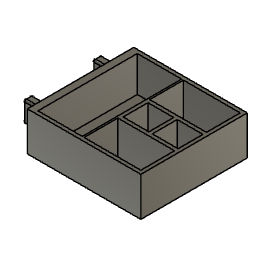
NP FW50 Charge Storagetray upright v4 (Autodesk Fusion 360 design; units mm, degrees)
Autodesk Fusion 360 part; units mm, degrees
note: some values were not read from the file. Chosen so that the rebuilt part matches the saved one: which face or edge a step refers to.
sketch "Skizze1" plane through (0, 0, 0) normal (0, 0, 1) x (1, 0, 0)
  line L0 (0, 0) -> (62, 0)
  line L1 (62, 0) -> (62, 60)
  line L2 (62, 60) -> (0, 60)
  line L3 (0, 60) -> (0, 0)
  line L4 (60, 2) -> (60, 58)
  line L5 (60, 58) -> (2, 58)
  line L6 (2, 58) -> (2, 2)
  line L7 (2, 2) -> (60, 2)
  line L8 (2, 58) -> (27, 58)
  line L9 (27, 58) -> (27, 2)
  line L10 (27, 2) -> (2, 2)
  line L11 (2, 2) -> (2, 58)
  line L12 (60, 58) -> (28, 58)
  line L13 (28, 58) -> (28, 39)
  line L14 (28, 39) -> (60, 39)
  line L15 (60, 39) -> (60, 58)
  line L16 (60, 2) -> (28, 2)
  line L17 (28, 2) -> (28, 21)
  line L18 (28, 21) -> (60, 21)
  line L19 (60, 21) -> (60, 2)
  line L20 (0, 60) -> (-2, 60)
  line L21 (-2, 60) -> (-2, 0)
  line L22 (-2, 0) -> (0, 0)
  line L23 (0, 0) -> (0, 60)
  dimension "d1" = 62
  dimension "d2" = 60
  dimension "d3" = -2
  dimension "d4" = 25
  dimension "d5" = 56
  dimension "d6" = 32
  dimension "d7" = 19
  dimension "d8" = 32
  dimension "d9" = 19
  dimension "d14" = 2
  dimension "d15" = 60
  constraint horizontal L0
  constraint vertical L1
  constraint horizontal L2
  constraint vertical L3
  constraint coincident L0.start L3.end
  constraint horizontal L8
  constraint vertical L9
  constraint horizontal L10
  constraint vertical L11
  constraint horizontal L12
  constraint vertical L13
  constraint horizontal L14
  constraint vertical L15
  constraint horizontal L16
  constraint vertical L17
  constraint horizontal L18
  constraint vertical L19
  constraint horizontal L20
  constraint vertical L21
  constraint horizontal L22
  constraint vertical L23
  measures "d1" distance of L0.start L0.end
  measures "d2" distance of L0.start L2.end
  measures "d4" distance of L5.end L8.end
  measures "d5" distance of L5.end L6.end
  measures "d6" distance of L4.end L12.end
  measures "d7" distance of L4.end L14.end
  measures "d8" distance of L4.start L16.end
  measures "d9" distance of L4.start L18.end
  measures "d14" distance of L2.end L20.end
  measures "d15" distance of L2.end L0.start
extrude "Extrusion1" add sketch "Skizze1" along normal blind 20 contours L0 L1 L2 L3 L23 | L3 L20 L21 L22 L23 | L4 L5 L7 L9 L13 L14 L17 L18
extrude "Extrusion2" add sketch "Skizze1" against normal blind 2 contours L0 L1 L2 L3 L23 | L3 L20 L21 L22 L23 | L4 L7 L16 L17 L18 L19 | L4 L5 L7 L9 L13 L14 L17 L18 | L4 L5 L12 L13 L14 L15 | L5 L6 L7 L8 L9 L10 L11
sketch "Skizze2" plane through (0, 0, 20) normal (0, 0, 1) x (-1, 0, 0)
  line L0 (-60, -58) -> (-60, -39)
  line L1 (-60, -39) -> (-28, -39)
  line L2 (-28, -39) -> (-28, -58)
  line L3 (-28, -58) -> (-60, -58)
  line L4 (-28, -21) -> (-60, -21)
  line L5 (-60, -21) -> (-60, -2)
  line L6 (-60, -2) -> (-28, -2)
  line L7 (-28, -2) -> (-28, -21)
  line L8 (-27, -2) -> (-2, -2)
  line L9 (-2, -2) -> (-2, -58)
  line L10 (-2, -58) -> (-27, -58)
  line L11 (-27, -58) -> (-27, -2)
  line L12 (2, 0) -> (-62, 0)
  line L13 (-62, 0) -> (-62, -60)
  line L14 (-62, -60) -> (2, -60)
  line L15 (2, -60) -> (2, 0)
  line L16 (-28, -23) -> (-60, -23)
  line L17 (-60, -37) -> (-28, -37)
  line L18 (-29, -58) -> (-29, -2)
  line L19 (-60, 0) -> (-60, -60)
  line L20 (-44.5, -30) -> (-44.5, -23)
  line L21 (-44.5, -30) -> (-44.5, -37)
  line L22 (-43.5, -30) -> (-43.5, -23)
  line L23 (-43.5, -30) -> (-43.5, -37)
  line L24 (-45.5, -30) -> (-45.5, -23)
  line L25 (-45.5, -30) -> (-45.5, -37)
  dimension "d16" = -2
  dimension "d17" = -2
  dimension "d18" = -2
  dimension "d19" = -2
  dimension "d20" = 1
  dimension "d21" = 1
  constraint coincident L16 L20.end
  constraint perpendicular L16 L20
  constraint coincident L17 L21.end
  constraint perpendicular L17 L21
extrude "Extrusion3" cut sketch "Skizze2" against normal blind 20 contours L16 L17 L19 L24 L25 | L16 L17 L18 L22 L23
sketch "Skizze3" plane through (-2, 0, 0) normal (-1, 0, 0) x (0, -1, 0)
  line L0 (0, -2) -> (0, 20)
  line L1 (0, 20) -> (-60, 20)
  line L2 (-60, 20) -> (-60, -2)
  line L3 (-60, -2) -> (0, -2)
  line L4 (-30, 20) -> (-30, -2)
  line L5 (-47, 20) -> (-47, -2)
  line L6 (-8, 20) -> (-8, -2)
  line L7 (-13, 20) -> (-13, -2)
  line L8 (-52, 20) -> (-52, -2)
  line L9 (0, 15.5) -> (-60, 15.5)
  line L10 (0, 11) -> (-60, 11)
  dimension "d26" = 17
  dimension "d27" = -22
  dimension "d28" = -17
  dimension "d29" = 22
  dimension "d30" = -4.5
  dimension "d31" = -9
  constraint midpoint L1 L4.start
  constraint midpoint L3 L4.end
  measures "d27" distance of L4
  measures "d29" distance of L4
extrude "Extrusion6" add sketch "Skizze3" along normal blind 5.5 contours L6 L7 L9 L10 | L5 L8 L9 L10
sketch "Skizze5" plane through (-7.5, 0, 0) normal (-1, 0, 0) x (0, -1, 0)
  line L0 (-52, 15.5) -> (-52, 11)
  line L1 (-52, 11) -> (-47, 11)
  line L2 (-47, 11) -> (-47, 15.5)
  line L3 (-47, 15.5) -> (-52, 15.5)
  line L4 (-52, 15.5) -> (-47, 15.5)
  line L5 (-47, 15.5) -> (-47, 3.5)
  line L6 (-47, 3.5) -> (-52, 3.5)
  line L7 (-52, 3.5) -> (-52, 15.5)
  line L8 (-8, 15.5) -> (-13, 15.5)
  line L9 (-13, 15.5) -> (-13, 3.5)
  line L10 (-13, 3.5) -> (-8, 3.5)
  line L11 (-8, 3.5) -> (-8, 15.5)
  dimension "d46" = 12
  dimension "d47" = 5
  dimension "d48" = 12
  constraint horizontal L4
  constraint vertical L5
  constraint horizontal L6
  constraint vertical L7
  constraint coincident L0.start L3.end
  constraint horizontal L8
  constraint vertical L9
  constraint horizontal L10
  constraint vertical L11
  measures "d46" distance of L0.start L6.end
  measures "d47" distance of L8.start L8.end
  measures "d48" distance of L8.start L10.end
extrude "Extrusion7" add sketch "Skizze5" along normal blind 5
fillet "Abrundung3" radius 1 12 edges at (-10, 47, 3.5) (-7.25, 47, 15.5) (-12.5, 47, 9.5) (-7.5, 47, 7.25) (-4.75, 47, 11) (-12.5, 49.5, 15.5) (-7.25, 52, 15.5) (-4.75, 52, 11) (-7.5, 52, 7.25) (-12.5, 52, 9.5) (-10, 52, 3.5) (-12.5, 49.5, 3.5)
fillet "Abrundung4" radius 1 12 edges at (-7.25, 13, 15.5) (-4.75, 13, 11) (-7.5, 13, 7.25) (-10, 13, 3.5) (-12.5, 10.5, 3.5) (-12.5, 13, 9.5) (-12.5, 10.5, 15.5) (-7.25, 8, 15.5) (-12.5, 8, 9.5) (-4.75, 8, 11) (-7.5, 8, 7.25) (-10, 8, 3.5)
extrude "Extrusion4" [rolled back] along distance 6 taper angle 0
sketch "Skizze4" plane through (-8, 0, 0) normal (-1, 0, 0) x (0, -1, 0)
  line L0 (-8, 11) -> (-8, 15.5)
  line L1 (-52, 11) -> (-8, 11)
  line L2 (-8, 15.5) -> (-52, 15.5)
  line L3 (-8, 11) -> (-4, 11)
  line L4 (-4, 11) -> (-4, -1)
  line L5 (-4, -1) -> (-8, -1)
  line L6 (-8, -1) -> (-8, 11)
  line L7 (-12.5, 15) -> (-8.5, 15)
  line L8 (-8.5, 15) -> (-8.5, 3)
  line L9 (-8.5, 3) -> (-12.5, 3)
  line L10 (-12.5, 3) -> (-12.5, 15)
  line L11 (-52, 15.5) -> (-52, 11)
  dimension "d34" = 4
  dimension "d35" = 12
  dimension "d36" = 4
  dimension "d37" = 12
  constraint horizontal L3
  constraint vertical L4
  constraint horizontal L5
  constraint vertical L6
  constraint coincident L0.start L1.end
  constraint horizontal L7
  constraint vertical L8
  constraint horizontal L9
  constraint vertical L10
  measures "d34" distance of L0.start L3.end
  measures "d35" distance of L0.start L5.end
  measures "d36" distance of L7.start L7.end
  measures "d37" distance of L7.start L9.end
extrude "Extrusion5" [rolled back] along distance 4 taper angle 0
